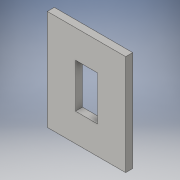
# Autodesk Inventor part: servo_mount
Saved by Autodesk Inventor 2016 (Build 200138000, 138)
## iProperties
Created: 2015-08-25
Part Number: servo_mount
Material: Generic
Document SubType Name: Modeling
Designer: chdsbd
Density: 1 g/cm^3
Appearance: Default
Author: chdsbd
Autodesk Inventor part; units mm, degrees
ref_plane "YZ Plane" through (0, 0, 0) normal (1, 0, 0) x (0, 1, 0)
ref_plane "XZ Plane" through (0, 0, 0) normal (0, 1, 0) x (-1, 0, 0)
ref_plane "XY Plane" through (0, 0, 0) normal (0, 0, 1) x (1, 0, 0)
sketch "Sketch1" plane through (0, 0, 0) normal (0, 0, 1) x (1, 0, 0)
  line L0 (-10, -20) -> (10, -20)
  line L1 (10, -20) -> (10, 20)
  line L2 (10, 20) -> (-10, 20)
  line L3 (-10, 20) -> (-10, -20)
  line L4 (-10, -20) -> (10, 20) construction
  line L5 (10, -20) -> (-10, 20) construction
  line L6 (-35.4, 45.4) -> (35.4, 45.4)
  line L7 (35.4, 45.4) -> (35.4, -45.4)
  line L8 (35.4, -45.4) -> (-35.4, -45.4)
  line L9 (-35.4, -45.4) -> (-35.4, 45.4)
  point P0 (0, 0)
  dimension "d0" = 20
  dimension "d1" = 40
  dimension "d6" = 25.4
  constraints: 20 end point, 4 parallel, 2 midpoint, 2 perpendicular, 1 horizontal, 3 other
  measures "d0" distance of L2.end L1.end
  measures "d1" distance of L1.end L0.end
  measures "d6" distance between parallel lines of L2 L6
extrude "Extrusion1" add sketch "Sketch1" along normal blind 6.35
body "Solid1"
